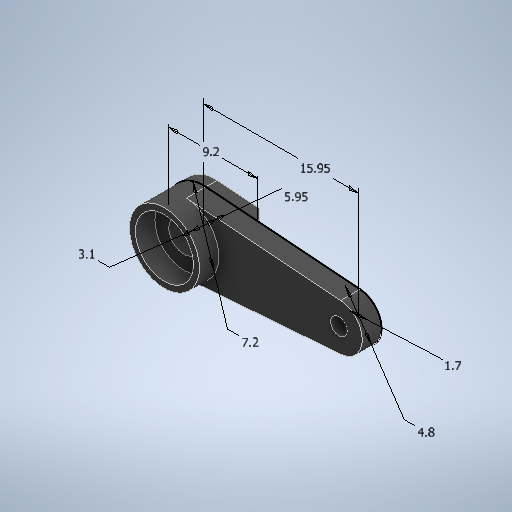
# Autodesk Inventor part: HalfServoArm
Saved by Autodesk Inventor 2025.1 (Build 291241000, 241)
## iProperties
Created: 2025-02-23
Part Number: HalfServoArm
Material: Generic
Document SubType Name: Modeling
Designer: 13156
Density: 1 g/cm^3
Appearance: Default
Author: 13156
Autodesk Inventor part; units mm, degrees
ref_plane "YZ Plane" through (0, 0, 0) normal (1, 0, 0) x (0, 1, 0)
ref_plane "XZ Plane" through (0, 0, 0) normal (0, 1, 0) x (-1, 0, 0)
ref_plane "XY Plane" through (0, 0, 0) normal (0, 0, 1) x (1, 0, 0)
sketch "Sketch1" plane through (0, 0, 0) normal (0, 0, 1) x (1, 0, 0)
  circle A0 centre (0, 0) radius 3.6
  line L0 (0, 0) -> (15.95, 0) construction
  circle A1 centre (15.95, 0) radius 2.4
  line L1 (0.2708, 3.5898) -> (16.1306, 2.3932)
  line L2 (0.2708, -3.5898) -> (16.1306, -2.3932)
  line L3 (5.6, 3.1877) -> (5.6, -3.1877)
  line L4 (0, 0) -> (-3.6, 0) construction
  circle A2 centre (0, 0) radius 1.55
  circle A3 centre (15.95, 0) radius 0.85
  circle A4 centre (0, 0) radius 2.975
  dimension "d0" = 7.2
  dimension "d1" = 4.8
  dimension "d2" = 15.95
  dimension "d5" = 9.2
  dimension "d6" = 3.1
  dimension "d7" = 1.7
  dimension "d10" = 5.95
  constraints: 11 end point, 5 centre point, 5 point on circle, 4 coincident, 4 tangent, 2 horizontal, 2 point on line, 1 vertical
  measures "d0" diameter of A0
  measures "d1" diameter of A1
  measures "d2" distance of L0.end point (0, 0)
  measures "d5" distance from line of L4.end L3
  measures "d6" diameter of A2
  measures "d7" diameter of A3
  measures "d10" diameter of A4
extrude "Extrusion1" add sketch "Sketch1" along normal blind 2 contours A0 | A0 L1 L3 L2 | L1 A1 L2 L3 | A1 | A4
extrude "Extrusion2" add sketch "Sketch1" against normal blind 1.15 contours A0 | A0 L1 L3 L2 | A4
extrude "Extrusion3" add sketch "Sketch1" along normal blind 4 contours A0
chamfer "Chamfer1" distance 1 angle 45 1 edges at (5.6, 0, -1.15)
body "Solid1"
